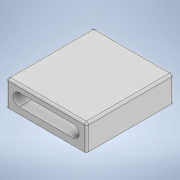
# Autodesk Inventor part: T5 SSD
Saved by Autodesk Inventor 2021 (Build 250183000, 183)
## iProperties
Created: 2022-08-23
Part Number: T5 SSD
Material: Generic
Document SubType Name: Modeling
Designer: cmzgt
Density: 1 g/cm^3
Appearance: Default
Author: cmzgt
Autodesk Inventor part; units mm, degrees
ref_plane "YZ Plane" through (0, 0, 0) normal (1, 0, 0) x (0, 1, 0)
ref_plane "XZ Plane" through (0, 0, 0) normal (0, 1, 0) x (-1, 0, 0)
ref_plane "XY Plane" through (0, 0, 0) normal (0, 0, 1) x (1, 0, 0)
sketch "Sketch1" plane through (0, 0, 0) normal (0, 0, 1) x (1, 0, 0)
  line L0 (34.925, -11.1125) -> (-34.925, -11.1125)
  line L1 (-34.925, -11.1125) -> (-34.925, 11.1125)
  line L2 (-34.925, 11.1125) -> (34.925, 11.1125)
  line L3 (34.925, 11.1125) -> (34.925, -11.1125)
  line L4 (34.925, -11.1125) -> (-34.925, 11.1125) construction
  line L5 (-34.925, -11.1125) -> (34.925, 11.1125) construction
  point P0 (0, 0)
  dimension "d0" = 69.85
  dimension "d1" = 22.225
  constraints: 12 end point, 2 midpoint, 2 parallel, 1 horizontal, 1 perpendicular
  measures "d0" distance of L1.end L2.end
  measures "d1" distance of L0.end L1.end
extrude "Extrusion1" add sketch "Sketch1" along normal blind 76.2
fillet "Fillet1" radius 1.905 8 edges at (34.925, 11.1125, 38.1) (-34.925, 11.1125, 38.1) (0, 11.1125, 0) (0, 11.1125, 76.2) (34.925, 0, 76.2) (-34.925, 0, 76.2) (34.925, 0, 0) (-34.925, 0, 0)
sketch "Sketch2" plane through (0, 0, 76.2) normal (0, 0, 1) x (1, 0, 0)
  line L0 (23.4, -5.35) -> (-23.4, -5.35)
  line L1 (-28.75, 0) -> (-28.75, 0)
  line L2 (-23.4, 5.35) -> (23.4, 5.35)
  line L3 (28.75, 0) -> (28.75, 0)
  line L4 (28.75, -5.35) -> (-28.75, 5.35) construction
  line L5 (-28.75, -5.35) -> (28.75, 5.35) construction
  arc A0 (-23.4, 5.35) -> (-28.75, 0) centre (-23.4, 0) ccw
  arc A1 (-28.75, 0) -> (-23.4, -5.35) centre (-23.4, 0) ccw
  arc A2 (28.75, 0) -> (23.4, 5.35) centre (23.4, 0) ccw
  arc A3 (23.4, -5.35) -> (28.75, 0) centre (23.4, 0) ccw
  point P0 (0, 0)
  point P1 (-28.75, 0)
  dimension "d5" = 57.5
  dimension "d6" = 10.7
  dimension "d9" = 5.35
  constraints: 12 end point, 8 point on circle, 8 point on line, 8 tangent, 4 centre point, 3 equal radius, 2 midpoint, 2 parallel, 1 horizontal, 1 perpendicular
  measures "d5" distance of L4.end L5.end
  measures "d6" distance of L5.start L4.end
  measures "d9" radius of A0
extrude "Extrusion2" cut sketch "Sketch2" against normal blind 69.85
sketch "Sketch3" plane through (0, 0, 0) normal (0, 0, -1) x (-1, 0, 0)
  line L0 (-23.4, -5.35) -> (23.4, -5.35) projected
  arc A0 (23.4, -5.35) -> (23.4, 5.35) centre (23.4, 0) ccw projected
  line L1 (23.4, 5.35) -> (-23.4, 5.35) projected
  arc A1 (-23.4, 5.35) -> (-23.4, -5.35) centre (-23.4, 0) ccw projected
  line L2 (7.62, -2.1403) -> (-7.62, -2.1403)
  line L3 (-7.62, -2.1403) -> (-7.62, 3.5747)
  line L4 (-7.62, 3.5747) -> (7.62, 3.5747)
  line L5 (7.62, 3.5747) -> (7.62, -2.1403)
  line L6 (7.62, -2.1403) -> (-7.62, 3.5747) construction
  line L7 (-7.62, -2.1403) -> (7.62, 3.5747) construction
  line L8 (33.02, 9.2075) -> (-33.02, 9.2075) projected
  line L9 (0, 9.2075) -> (0, -11.1125)
  line L10 (33.02, -11.1125) -> (-33.02, -11.1125) projected
  point P0 (0, 0)
  point P1 (0, 0.7172)
  dimension "d10" = 15.24
  dimension "d11" = 5.715
  dimension "d13" = 4.6328
  constraints: 14 end point, 4 midpoint, 2 parallel, 1 horizontal, 1 perpendicular, 1 point on line, 1 vertical
  measures "d10" distance of L3.end L4.end
  measures "d11" distance of L4.end L2.start
  measures "d13" distance from line of L1 point (0, 0.717)
extrude "Extrusion3" cut sketch "Sketch3" against normal through all contours L9 L4 L5 L2 | L2 L3 L4 L9
body "Solid1"
